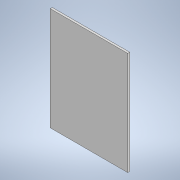
# Autodesk Inventor part: 6080_pcb
Saved by Autodesk Inventor 2022.1 (Build 261234020, 234B)
## iProperties
Created: 2022-02-07
Part Number: 6080_pcb
Material: Generic
Document SubType Name: Modeling
Designer: kee
Density: 1 g/cm^3
Appearance: Default
Mass: 7.68 g
Surface Area: 100.48 cm^2
Volume: 7.68 cm^3
Author: kee
Autodesk Inventor part; units mm, degrees
ref_plane "YZ Plane" through (0, 0, 0) normal (1, 0, 0) x (0, 1, 0)
ref_plane "XZ Plane" through (0, 0, 0) normal (0, 1, 0) x (-1, 0, 0)
ref_plane "XY Plane" through (0, 0, 0) normal (0, 0, 1) x (1, 0, 0)
sketch "Sketch1" plane through (0, 0, 0) normal (0, 0, 1) x (1, 0, 0)
  line L0 (-30, 40) -> (30, 40)
  line L1 (30, 40) -> (30, -40)
  line L2 (30, -40) -> (-30, -40)
  line L3 (-30, -40) -> (-30, 40)
  point P0 (0, 0)
  dimension "d0" = 60
  dimension "d1" = 30
  dimension "d2" = 80
  dimension "d3" = 40
  constraints: 8 end point, 2 parallel, 1 horizontal, 1 perpendicular
  measures "d0" distance of L0.end L0.start
  measures "d1" horizontal distance of point (0, 0) L0.start
  measures "d2" distance between parallel lines of L2 L0
  measures "d3" vertical distance of point (0, 0) L0.end
extrude "Extrusion1" add sketch "Sketch1" along normal blind 1.6
equation "\"d1\" = 0.5 * d0"
equation "\"d3\" = 0.5 * d2"
body "Solid1"
